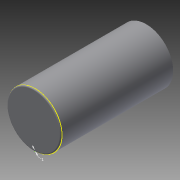
# Autodesk Inventor part: Dalek Light 2
Saved by Autodesk Inventor 2015 (Build 190159000, 159)
## iProperties
Created: 2014-09-01
Part Number: Dalek Light 2
Material: Generic
Document SubType Name: Modeling
Designer: Chris
Density: 1 g/cm^3
Appearance: Default
Author: Chris
Autodesk Inventor part; units mm, degrees
ref_plane "YZ Plane" through (0, 0, 0) normal (1, 0, 0) x (0, 1, 0)
ref_plane "XZ Plane" through (0, 0, 0) normal (0, 1, 0) x (-1, 0, 0)
ref_plane "XY Plane" through (0, 0, 0) normal (0, 0, 1) x (1, 0, 0)
sketch "Sketch1" plane through (0, 0, 0) normal (0, 1, 0) x (-1, 0, 0)
  circle A0 centre (0, 0) radius 22.5
  circle A1 centre (0, 0) radius 23
  dimension "d0" = 45
  dimension "d1" = 46
  constraints: 2 centre point, 2 coincident
  measures "d0" diameter of A0
  measures "d1" diameter of A1
extrude "Extrusion1" add sketch "Sketch1" along normal blind 95
sketch "Sketch2" plane through (0, 0, 0) normal (0, -1, 0) x (1, 0, 0)
  circle A0 centre (0, 0) radius 23 projected
  circle A1 centre (0, -23) radius 0.5
  dimension "d8" = 1
  constraints: 1 centre point, 1 vertical alignment, 1 other
  measures "d8" diameter of A1
sketch "Sketch3" plane through (0, 0, 0) normal (0, -1, 0) x (1, 0, 0)
  circle A0 centre (0, 0) radius 23
  dimension "d4" = 46
  constraints: 1 centre point, 1 coincident
  measures "d4" diameter of A0
extrude "Extrusion2" add sketch "Sketch3" along normal blind 1
fillet "Fillet1" radius 1 1 edges at (-23, -1, 0)
body "Solid1"
